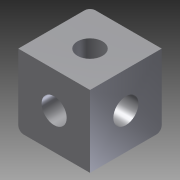
# Autodesk Inventor part: Corner Profile
Saved by Autodesk Inventor 2012 (Build 160160000, 160)
## iProperties
Created: 2013-02-22
Part Number: Corner Profile
Material: Default
Document SubType Name: Modeling
Designer: mce
Density: 1 g/cm^3
Mass: 6.1476 g
Surface Area: 30.3238 cm^2
Volume: 6.1476 cm^3
Author: mce
Autodesk Inventor part; units mm, degrees
ref_plane "YZ Plane" through (0, 0, 0) normal (1, 0, 0) x (0, 1, 0)
ref_plane "XZ Plane" through (0, 0, 0) normal (0, 1, 0) x (-1, 0, 0)
ref_plane "XY Plane" through (0, 0, 0) normal (0, 0, 1) x (1, 0, 0)
sketch "Sketch1" plane through (0, 0, 0) normal (0, 0, 1) x (1, 0, 0)
  line L0 (0, 0) -> (20, 0)
  line L1 (20, 0) -> (20, 20)
  line L2 (20, 20) -> (0, 20)
  line L3 (0, 20) -> (0, 0)
  circle A0 centre (10, 10) radius 3.5
  dimension "d0" = 20
  dimension "d1" = 20
  dimension "d2" = 7
  constraints: 8 end point, 1 centre point
  measures "d0" distance of L0.start L0.end
  measures "d1" distance of L2.end L0.start
  measures "d2" diameter of A0
extrude "Extrusion1" add sketch "Sketch1" along normal blind 20
sketch "Sketch2" plane through (20, 0, 0) normal (1, 0, 0) x (0, 0, -1)
  circle A0 centre (-10, 10) radius 3.5
  dimension "d5" = 7
  constraints: 1 centre point
  measures "d5" diameter of A0
extrude "Extrusion2" cut sketch "Sketch2" against normal blind 20
sketch "Sketch3" plane through (0, 0, 0) normal (0, -1, 0) x (1, 0, 0)
  circle A0 centre (10, 10) radius 3.5
  dimension "d8" = 7
  constraints: 1 centre point
  measures "d8" diameter of A0
extrude "Extrusion3" cut sketch "Sketch3" against normal blind 20
fillet "Fillet1" radius 1.5 3 edges at (0, 10, 0) (0, 20, 10) (10, 20, 0)
body "Solid1"
